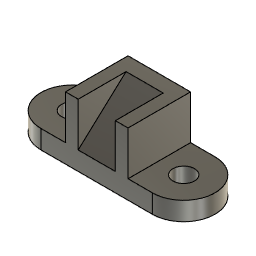
A2 Shape (Autodesk Fusion 360 design; units mm, degrees)
Autodesk Fusion 360 part; units mm, degrees
note: some values were not read from the file. Set by a fixed rule: which sketch regions a step uses.
sketch "Sketch1" plane through (0, 0, 0) normal (0, 0, 1) x (1, 0, 0)
  line L0 (57, 32) -> (-57, 32)
  line L1 (-57, 32) -> (-57, -32)
  line L2 (-57, -32) -> (57, -32)
  line L3 (57, -32) -> (57, 32)
  line L4 (57, 32) -> (-57, -32) construction
  line L5 (-57, 32) -> (57, -32) construction
  line L6 (-32, 32) -> (-32, -32) construction
  line L7 (32, 32) -> (32, -32) construction
  circle A0 centre (57, 0) radius 11
  circle A1 centre (-57, 0) radius 11
  circle A2 centre (-57, 0) radius 32
  circle A3 centre (57, 0) radius 32
  dimension "d1" = 114
  dimension "d2" = 64
  dimension "d3" = 64
  dimension "d4" = 25
  dimension "d5" = 22
  dimension "d6" = 22
  dimension "d7" = 32
  dimension "d8" = 32
  constraint horizontal L0
  constraint perpendicular L0 L1
  constraint parallel L0 L2
  constraint parallel L1 L3
  constraint coincident L4 origin
  constraint coincident L5 origin
  constraint coincident L0 L6.start
  constraint coincident L2 L6.end
  constraint perpendicular L2 L6
  constraint coincident L0 L7.start
  constraint coincident L2 L7.end
  constraint perpendicular L2 L7
  constraint midpoint L3 A0.centre
  constraint midpoint L1 A1.centre
  constraint concentric A1 A2
  constraint concentric A0 A3
  measures "d1" distance of L1.end L2.end
  measures "d2" distance of L0.end L1.end
  measures "d3" distance of L6 L7
  measures "d4" distance of L3 L7
  measures "d5" diameter of A0
  measures "d6" diameter of A1
  measures "d7" radius of A2
  measures "d8" radius of A3
extrude "Extrude1" add sketch "Sketch1" along normal blind 19 contours L0 L2 A2 A3 | L3 A0 A3 | L3 A0 A3 | L1 A1 A2 | L1 A1 A2
sketch "Sketch2" plane through (0, 0, 0) normal (1, 0, 0) x (0, 1, 0)
  line L0 (-32, 19) -> (32, 19)
  line L1 (32, 19) -> (32, 64)
  line L2 (32, 64) -> (17, 64)
  line L3 (17, 64) -> (-32, 19)
  dimension "d11" = 45
  dimension "d13" = 15
  constraint horizontal L0
  constraint perpendicular L0 L1
  constraint perpendicular L1 L2
  measures "d11" distance of L0.end L1.end
  measures "d13" distance of L1.end L2.end
extrude "Extrude2" add sketch "Sketch2" along normal mid plane 38
sketch "Sketch3" plane through (19, 0, 0) normal (1, 0, 0) x (0, 1, 0)
  line L0 (17, 64) -> (-32, 19)
  line L1 (-32, 19) -> (32, 19)
  line L2 (32, 19) -> (32, 64)
  line L3 (32, 64) -> (17, 64)
  line L4 (-32, 19) -> (32, 19)
  line L5 (32, 19) -> (32, 64)
  line L6 (32, 64) -> (-32, 64)
  line L7 (-32, 64) -> (-32, 19)
  constraint coincident L0.end L1.start
  constraint coincident L1.end L2.start
  constraint coincident L2.end L3.start
  constraint perpendicular L5 L6
  constraint perpendicular L4 L7
extrude "Extrude3" add sketch "Sketch3" along normal blind 13
sketch "Sketch4" plane through (-19, 0, 0) normal (-1, 0, 0) x (0, -1, 0)
  line L0 (32, 19) -> (-17, 64)
  line L1 (-17, 64) -> (-32, 64)
  line L2 (-32, 64) -> (-32, 19)
  line L3 (-32, 19) -> (32, 19)
  line L4 (-32, 64) -> (32, 64)
  line L5 (32, 64) -> (32, 19)
  line L6 (32, 19) -> (-32, 19)
  line L7 (-32, 64) -> (-32, 19)
  constraint coincident L1.end L2.start
  constraint perpendicular L2 L4
  constraint coincident L0.start L3.end
  constraint perpendicular L1 L5
  constraint coincident L2.end L3.start
extrude "Extrude4" add sketch "Sketch4" along normal blind 13
